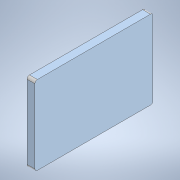
# Autodesk Inventor part: Part121
Saved by Autodesk Inventor 2022 (Build 260153070, 153G)
## iProperties
Created: 2021-07-11
Part Number: Part121
Material: Generic
Document SubType Name: Modeling
Designer: sachin
Density: 1 g/cm^3
Appearance: Default
Author: sachin
Autodesk Inventor part; units mm, degrees
ref_plane "YZ Plane" through (0, 0, 0) normal (1, 0, 0) x (0, 1, 0)
ref_plane "XZ Plane" through (0, 0, 0) normal (0, 1, 0) x (-1, 0, 0)
ref_plane "XY Plane" through (0, 0, 0) normal (0, 0, 1) x (1, 0, 0)
sketch "Sketch1" plane through (0, 0, 0) normal (1, 0, 0) x (0, 1, 0)
  line L0 (54.153, 111.5998) -> (-47.447, 111.5998)
  line L1 (-47.447, 111.5998) -> (-47.447, -40.8002)
  line L2 (-47.447, -40.8002) -> (54.153, -40.8002)
  line L3 (54.153, -40.8002) -> (54.153, 111.5998)
  point P0 (0, 0)
  dimension "d0" = 152.4
  dimension "d1" = 101.6
  constraints: 8 end point, 2 parallel, 1 horizontal, 1 perpendicular
  measures "d0" distance of L2.end L0.start
  measures "d1" distance of L1.end L2.end
extrude "Extrusion1" add sketch "Sketch1" along normal blind 10.16
fillet "Fillet1" radius 3.175 4 edges at (5.08, 54.153, 111.5998) (5.08, 54.153, -40.8002) (5.08, -47.447, -40.8002) (5.08, -47.447, 111.5998)
body "Solid1"
